Autodesk Inventor part; units mm, degrees
(part 3 of 4)
  line L1598 (-32.17063, 1.012888) -> (-32.17063, -0.001143)
  line L1599 (-32.17063, -0.001143) -> (-32.17063, -0.963359)
  line L1600 (-32.17063, -0.963359) -> (-31.94224, -3.850005)
  line L1601 (-31.94224, -3.850005) -> (-31.272499, -7.565517)
  line L1602 (-31.272499, -7.565517) -> (-30.188344, -11.120628)
  line L1603 (-30.188344, -11.120628) -> (-28.715551, -14.490001)
  line L1604 (-28.715551, -14.490001) -> (-26.883112, -17.647539)
  line L1605 (-26.883112, -17.647539) -> (-24.714784, -20.565161)
  line L1606 (-24.714784, -20.565161) -> (-22.239465, -23.217188)
  line L1607 (-22.239465, -23.217188) -> (-20.201363, -25.028976)
  line L1608 (-20.201363, -25.028976) -> (-19.480987, -25.578797)
  line L1609 (-19.480987, -25.578797) -> (-19.035522, -24.981427)
  line L1610 (-19.035522, -24.981427) -> (-19.739362, -24.443988)
  line L1611 (-19.739362, -24.443988) -> (-21.728906, -22.674586)
  line L1612 (-21.728906, -22.674586) -> (-24.146332, -20.08352)
  line L1613 (-24.146332, -20.08352) -> (-26.262997, -17.234154)
  line L1614 (-26.262997, -17.234154) -> (-28.05202, -14.151102)
  line L1615 (-28.05202, -14.151102) -> (-29.489667, -10.861358)
  line L1616 (-29.489667, -10.861358) -> (-30.547989, -7.388733)
  line L1617 (-30.547989, -7.388733) -> (-31.202243, -3.759899)
  line L1618 (-31.202243, -3.759899) -> (-31.425471, -0.940499)
  line L1619 (-31.425471, -0.940499) -> (-31.425471, -0.001143)
  circle A0 centre (0, 0) radius 38.1
  circle A1 centre (0, 0) radius 38.1
  line L1620 (0, -38.1) -> (0, -50.8)
  line L1621 (0, -38.1) -> (12.7, -38.1) construction
  point P0 (0, 45.086841)
  dimension "d32" = 76.2
  dimension "d33" = 12.7
  dimension "d34" = 90
  constraints: 3244 end point, 1 horizontal, 1 perpendicular, 1 vertical, 1 vertical alignment, 1 other
  measures "d32" distance of L125.end L89.end
  measures "d33" distance of L1620.start L1620.end
  measures "d34" angle of L1620 L1621
sketch "Sketch3 outline for Extrusion2" plane through (0, -45.086841, 3.175) normal (0, 0, 1) x (1, 0, 0)
  circle A0 centre (0, 0) radius 38.1
  line L0 (0.918972, -35.952322) -> (-0.919924, -35.952322)
  line L1 (-0.919924, -35.952322) -> (-3.676459, -35.766299)
  line L2 (-3.676459, -35.766299) -> (-7.246239, -35.221621)
  line L3 (-7.246239, -35.221621) -> (-10.691812, -34.335872)
  line L4 (-10.691812, -34.335872) -> (-13.995083, -33.126655)
  line L5 (-13.995083, -33.126655) -> (-17.136999, -31.612542)
  line L6 (-17.136999, -31.612542) -> (-20.101103, -29.812145)
  line L7 (-20.101103, -29.812145) -> (-22.868896, -27.741982)
  line L8 (-22.868896, -27.741982) -> (-25.421692, -25.421692)
  line L9 (-25.421692, -25.421692) -> (-27.74301, -22.868896)
  line L10 (-27.74301, -22.868896) -> (-29.812145, -20.101103)
  line L11 (-29.812145, -20.101103) -> (-31.612542, -17.136999)
  line L12 (-31.612542, -17.136999) -> (-33.126655, -13.99394)
  line L13 (-33.126655, -13.99394) -> (-34.335872, -10.690669)
  line L14 (-34.335872, -10.690669) -> (-35.221621, -7.246239)
  line L15 (-35.221621, -7.246239) -> (-35.766299, -3.67646)
  line L16 (-35.766299, -3.67646) -> (-35.951293, -0.919925)
  line L17 (-35.951293, -0.919925) -> (-35.951293, 0.918972)
  line L18 (-35.951293, 0.918972) -> (-35.766299, 3.675316)
  line L19 (-35.766299, 3.675316) -> (-35.221621, 7.245096)
  line L20 (-35.221621, 7.245096) -> (-34.335872, 10.689717)
  line L21 (-34.335872, 10.689717) -> (-33.126655, 13.992987)
  line L22 (-33.126655, 13.992987) -> (-31.612542, 17.136046)
  line L23 (-31.612542, 17.136046) -> (-29.812145, 20.100036)
  line L24 (-29.812145, 20.100036) -> (-27.74301, 22.868001)
  line L25 (-27.74301, 22.868001) -> (-25.421692, 25.420701)
  line L26 (-25.421692, 25.420701) -> (-22.868896, 27.740991)
  line L27 (-22.868896, 27.740991) -> (-20.101103, 29.811155)
  line L28 (-20.101103, 29.811155) -> (-17.136999, 31.61157)
  line L29 (-17.136999, 31.61157) -> (-13.995083, 33.125664)
  line L30 (-13.995083, 33.125664) -> (-10.691812, 34.334958)
  line L31 (-10.691812, 34.334958) -> (-7.246239, 35.220592)
  line L32 (-7.246239, 35.220592) -> (-3.676459, 35.765232)
  line L33 (-3.676459, 35.765232) -> (-0.919924, 35.950207)
  line L34 (-0.919924, 35.950207) -> (0.918972, 35.950207)
  line L35 (0.918972, 35.950207) -> (3.675317, 35.765232)
  line L36 (3.675317, 35.765232) -> (7.245096, 35.220592)
  line L37 (7.245096, 35.220592) -> (10.69067, 34.334958)
  line L38 (10.69067, 34.334958) -> (13.99413, 33.125664)
  line L39 (13.99413, 33.125664) -> (17.136999, 31.61157)
  line L40 (17.136999, 31.61157) -> (20.101179, 29.811155)
  line L41 (20.101179, 29.811155) -> (22.868954, 27.740991)
  line L42 (22.868954, 27.740991) -> (25.421653, 25.420701)
  line L43 (25.421653, 25.420701) -> (27.742134, 22.868001)
  line L44 (27.742134, 22.868001) -> (29.812107, 20.100036)
  line L45 (29.812107, 20.100036) -> (31.612332, 17.136046)
  line L46 (31.612332, 17.136046) -> (33.126617, 13.992987)
  line L47 (33.126617, 13.992987) -> (34.33572, 10.689717)
  line L48 (34.33572, 10.689717) -> (35.221545, 7.245096)
  line L49 (35.221545, 7.245096) -> (35.766375, 3.675316)
  line L50 (35.766375, 3.675316) -> (35.952303, 0.918972)
  line L51 (35.952303, 0.918972) -> (35.952303, -0.919925)
  line L52 (35.952303, -0.919925) -> (35.766375, -3.67646)
  line L53 (35.766375, -3.67646) -> (35.221545, -7.246239)
  line L54 (35.221545, -7.246239) -> (34.33572, -10.690669)
  line L55 (34.33572, -10.690669) -> (33.126617, -13.99394)
  line L56 (33.126617, -13.99394) -> (31.612332, -17.136999)
  line L57 (31.612332, -17.136999) -> (29.812107, -20.101103)
  line L58 (29.812107, -20.101103) -> (27.742134, -22.868896)
  line L59 (27.742134, -22.868896) -> (25.421653, -25.421692)
  line L60 (25.421653, -25.421692) -> (22.868954, -27.741982)
  line L61 (22.868954, -27.741982) -> (20.101179, -29.812145)
  line L62 (20.101179, -29.812145) -> (17.136999, -31.612542)
  line L63 (17.136999, -31.612542) -> (13.99413, -33.126655)
  line L64 (13.99413, -33.126655) -> (10.69067, -34.335872)
  line L65 (10.69067, -34.335872) -> (7.245096, -35.221621)
  line L66 (7.245096, -35.221621) -> (3.675317, -35.766299)
  line L67 (3.675317, -35.766299) -> (0.918972, -35.952322)
  line L68 (-29.911357, 16.940403) -> (-28.194667, 16.119919)
  line L69 (-28.194667, 16.119919) -> (-28.483008, 15.517368)
  line L70 (-28.483008, 15.517368) -> (-28.579134, 15.56385)
  line L71 (-28.579134, 15.56385) -> (-29.008045, 15.702534)
  line L72 (-29.008045, 15.702534) -> (-29.370814, 15.721012)
  line L73 (-29.370814, 15.721012) -> (-29.433869, 15.706534)
  line L74 (-29.433869, 15.706534) -> (-29.496906, 15.693199)
  line L75 (-29.496906, 15.693199) -> (-29.769759, 15.530703)
  line L76 (-29.769759, 15.530703) -> (-29.98992, 15.24762)
  line L77 (-29.98992, 15.24762) -> (-30.025048, 15.172182)
  line L78 (-30.025048, 15.172182) -> (-30.05709, 15.103983)
  line L79 (-30.05709, 15.103983) -> (-27.229365, 13.752195)
  line L80 (-27.229365, 13.752195) -> (-27.191094, 13.734478)
  line L81 (-27.191094, 13.734478) -> (-26.930661, 13.63218)
  line L82 (-26.930661, 13.63218) -> (-26.916202, 13.629132)
  line L83 (-26.916202, 13.629132) -> (-26.902753, 13.628179)
  line L84 (-26.902753, 13.628179) -> (-26.792149, 13.661136)
  line L85 (-26.792149, 13.661136) -> (-26.7839, 13.669518)
  line L86 (-26.7839, 13.669518) -> (-26.773556, 13.678662)
  line L87 (-26.773556, 13.678662) -> (-26.665028, 13.817346)
  line L88 (-26.665028, 13.817346) -> (-26.653674, 13.834872)
  line L89 (-26.653674, 13.834872) -> (-26.642301, 13.85335)
  line L90 (-26.642301, 13.85335) -> (-26.462469, 14.188249)
  line L91 (-26.462469, 14.188249) -> (-26.437666, 14.237017)
  line L92 (-26.437666, 14.237017) -> (-25.867157, 13.96384)
  line L93 (-25.867157, 13.96384) -> (-27.129105, 11.324463)
  line L94 (-27.129105, 11.324463) -> (-27.699595, 11.597259)
  line L95 (-27.699595, 11.597259) -> (-27.68306, 11.632311)
  line L96 (-27.68306, 11.632311) -> (-27.552834, 11.935015)
  line L97 (-27.552834, 11.935015) -> (-27.542509, 11.961114)
  line L98 (-27.542509, 11.961114) -> (-27.533194, 11.987974)
  line L99 (-27.533194, 11.987974) -> (-27.474272, 12.213145)
  line L100 (-27.474272, 12.213145) -> (-27.471186, 12.231624)
  line L101 (-27.471186, 12.231624) -> (-27.470157, 12.243054)
  line L102 (-27.470157, 12.243054) -> (-27.514601, 12.347638)
  line L103 (-27.514601, 12.347638) -> (-27.524926, 12.356782)
  line L104 (-27.524926, 12.356782) -> (-27.53527, 12.367069)
  line L105 (-27.53527, 12.367069) -> (-27.772976, 12.503658)
  line L106 (-27.772976, 12.503658) -> (-27.8102, 12.521184)
  line L107 (-27.8102, 12.521184) -> (-27.898039, 12.563475)
  line L108 (-27.898039, 12.563475) -> (-30.645144, 13.877163)
  line L109 (-30.645144, 13.877163) -> (-30.676158, 13.812012)
  line L110 (-30.676158, 13.812012) -> (-30.712334, 13.736574)
  line L111 (-30.712334, 13.736574) -> (-30.750586, 13.066966)
  line L112 (-30.750586, 13.066966) -> (-30.721649, 13.007911)
  line L113 (-30.721649, 13.007911) -> (-30.693722, 12.949999)
  line L114 (-30.693722, 12.949999) -> (-30.075683, 12.431268)
  line L115 (-30.075683, 12.431268) -> (-29.980604, 12.385929)
  line L116 (-29.980604, 12.385929) -> (-30.26584, 11.788521)
  line L117 (-30.26584, 11.788521) -> (-31.98255, 12.609957)
  line L118 (-31.98255, 12.609957) -> (-29.911357, 16.940403)
  line L119 (-9.504426, -27.822582) -> (-10.266045, -29.566152)
  line L120 (-10.266045, -29.566152) -> (-10.876788, -29.29951)
  line L121 (-10.876788, -29.29951) -> (-10.834497, -29.202355)
  line L122 (-10.834497, -29.202355) -> (-10.711434, -28.768281)
  line L123 (-10.711434, -28.768281) -> (-10.704195, -28.404483)
  line L124 (-10.704195, -28.404483) -> (-10.719816, -28.342457)
  line L125 (-10.719816, -28.342457) -> (-10.736199, -28.279401)
  line L126 (-10.736199, -28.279401) -> (-10.90803, -28.01173)
  line L127 (-10.90803, -28.01173) -> (-11.199305, -27.802942)
  line L128 (-11.199305, -27.802942) -> (-11.274742, -27.769871)
  line L129 (-11.274742, -27.769871) -> (-11.344084, -27.739905)
  line L130 (-11.344084, -27.739905) -> (-12.598718, -30.612074)
  line L131 (-12.598718, -30.612074) -> (-12.616243, -30.650307)
  line L132 (-12.616243, -30.650307) -> (-12.708255, -30.915959)
  line L133 (-12.708255, -30.915959) -> (-12.709398, -30.930399)
  line L134 (-12.709398, -30.930399) -> (-12.711303, -30.943848)
  line L135 (-12.711303, -30.943848) -> (-12.674155, -31.053405)
  line L136 (-12.674155, -31.053405) -> (-12.664821, -31.061654)
  line L137 (-12.664821, -31.061654) -> (-12.655486, -31.070969)
  line L138 (-12.655486, -31.070969) -> (-12.51604, -31.174315)
  line L139 (-12.51604, -31.174315) -> (-12.496419, -31.185688)
  line L140 (-12.496419, -31.185688) -> (-12.47775, -31.196013)
  line L141 (-12.47775, -31.196013) -> (-12.136755, -31.364511)
  line L142 (-12.136755, -31.364511) -> (-12.087034, -31.388266)
  line L143 (-12.087034, -31.388266) -> (-12.339256, -31.967043)
  line L144 (-12.339256, -31.967043) -> (-15.021306, -30.797068)
  line L145 (-15.021306, -30.797068) -> (-14.769084, -30.217262)
  line L146 (-14.769084, -30.217262) -> (-14.734032, -30.23174)
  line L147 (-14.734032, -30.23174) -> (-14.425994, -30.351622)
  line L148 (-14.425994, -30.351622) -> (-14.399133, -30.360937)
  line L149 (-14.399133, -30.360937) -> (-14.373225, -30.369186)
  line L150 (-14.373225, -30.369186) -> (-14.145958, -30.420888)
  line L151 (-14.145958, -30.420888) -> (-14.126337, -30.422964)
  line L152 (-14.126337, -30.422964) -> (-14.114907, -30.423993)
  line L153 (-14.114907, -30.423993) -> (-14.012608, -30.376444)
  line L154 (-14.012608, -30.376444) -> (-14.003274, -30.3661)
  line L155 (-14.003274, -30.3661) -> (-13.993939, -30.354746)
  line L156 (-13.993939, -30.354746) -> (-13.865733, -30.111859)
  line L157 (-13.865733, -30.111859) -> (-13.84935, -30.074654)
  line L158 (-13.84935, -30.074654) -> (-13.809916, -29.984719)
  line L159 (-13.809916, -29.984719) -> (-12.591478, -27.195247)
  line L160 (-12.591478, -27.195247) -> (-12.656629, -27.16631)
  line L161 (-12.656629, -27.16631) -> (-12.734163, -27.13221)
  line L162 (-12.734163, -27.13221) -> (-13.405866, -27.117732)
  line L163 (-13.405866, -27.117732) -> (-13.462825, -27.148746)
  line L164 (-13.462825, -27.148746) -> (-13.520547, -27.178711)
  line L165 (-13.520547, -27.178711) -> (-14.017752, -27.812257)
  line L166 (-14.017752, -27.812257) -> (-14.05909, -27.909412)
  line L167 (-14.05909, -27.909412) -> (-14.66469, -27.645855)
  line L168 (-14.66469, -27.645855) -> (-13.903071, -25.901256)
  line L169 (-13.903071, -25.901256) -> (-9.504426, -27.822582)
  line L170 (5.837492, -31.82855) -> (6.61035, -31.72728)
  line L171 (6.61035, -31.72728) -> (6.626923, -31.895739)
  line L172 (6.626923, -31.895739) -> (6.568059, -32.634688)
  line L173 (6.568059, -32.634688) -> (6.313742, -33.231049)
  line L174 (6.313742, -33.231049) -> (6.234303, -33.329213)
  line L175 (6.234303, -33.329213) -> (6.153722, -33.426368)
  line L176 (6.153722, -33.426368) -> (5.610034, -33.802587)
  line L177 (5.610034, -33.802587) -> (4.875276, -34.029968)
  line L178 (4.875276, -34.029968) -> (4.700587, -34.053723)
  line L179 (4.700587, -34.053723) -> (4.502087, -34.079574)
  line L180 (4.502087, -34.079574) -> (3.60807, -34.017566)
  line L181 (3.60807, -34.017566) -> (2.845308, -33.700269)
  line L182 (2.845308, -33.700269) -> (2.711958, -33.59898)
  line L183 (2.711958, -33.59898) -> (2.578608, -33.496682)
  line L184 (2.578608, -33.496682) -> (2.072259, -32.844505)
  line L185 (2.072259, -32.844505) -> (1.781747, -32.000114)
  line L186 (1.781747, -32.000114) -> (1.756029, -31.802699)
  line L187 (1.756029, -31.802699) -> (1.742504, -31.703486)
  line L188 (1.742504, -31.703486) -> (1.777746, -30.802269)
  line L189 (1.777746, -30.802269) -> (1.79832, -30.720621)
  line L190 (1.79832, -30.720621) -> (1.817941, -30.638953)
  line L191 (1.817941, -30.638953) -> (2.190941, -29.877258)
  line L192 (2.190941, -29.877258) -> (2.245805, -29.806944)
  line L193 (2.245805, -29.806944) -> (2.298764, -29.739774)
  line L194 (2.298764, -29.739774) -> (2.906268, -29.215804)
  line L195 (2.906268, -29.215804) -> (2.97542, -29.178561)
  line L196 (2.97542, -29.178561) -> (3.043809, -29.140328)
  line L197 (3.043809, -29.140328) -> (3.861245, -28.891249)
  line L198 (3.861245, -28.891249) -> (3.956304, -28.879876)
  line L199 (3.956304, -28.879876) -> (4.022408, -28.870599)
  line L200 (4.022408, -28.870599) -> (4.659059, -28.884029)
  line L201 (4.659059, -28.884029) -> (4.720209, -28.896412)
  line L202 (4.720209, -28.896412) -> (4.780979, -28.907784)
  line L203 (4.780979, -28.907784) -> (5.382768, -29.13105)
  line L204 (5.382768, -29.13105) -> (5.442395, -29.164121)
  line L205 (5.442395, -29.164121) -> (5.537645, -28.756908)
  line L206 (5.537645, -28.756908) -> (6.206299, -28.66905)
  line L207 (6.206299, -28.66905) -> (6.469952, -30.662728)
  line L208 (6.469952, -30.662728) -> (5.753671, -30.757806)
  line L209 (5.753671, -30.757806) -> (5.731955, -30.651374)
  line L210 (5.731955, -30.651374) -> (5.564505, -30.19867)
  line L211 (5.564505, -30.19867) -> (5.315522, -29.854493)
  line L212 (5.315522, -29.854493) -> (5.253228, -29.801801)
  line L213 (5.253228, -29.801801) -> (5.190363, -29.74909)
  line L214 (5.190363, -29.74909) -> (4.837938, -29.581659)
  line L215 (4.837938, -29.581659) -> (4.431792, -29.543426)
  line L216 (4.431792, -29.543426) -> (4.342829, -29.555808)
  line L217 (4.342829, -29.555808) -> (4.244721, -29.56821)
  line L218 (4.244721, -29.56821) -> (3.835337, -29.747032)
  line L219 (3.835337, -29.747032) -> (3.533585, -30.077759)
  line L220 (3.533585, -30.077759) -> (3.490151, -30.166628)
  line L221 (3.490151, -30.166628) -> (3.445574, -30.255534)
  line L222 (3.445574, -30.255534) -> (3.320796, -30.787791)
  line L223 (3.320796, -30.787791) -> (3.322892, -31.437872)
  line L224 (3.322892, -31.437872) -> (3.342513, -31.585662)
  line L225 (3.342513, -31.585662) -> (3.362135, -31.735528)
  line L226 (3.362135, -31.735528) -> (3.528441, -32.372198)
  line L227 (3.528441, -32.372198) -> (3.785997, -32.854849)
  line L228 (3.785997, -32.854849) -> (3.850958, -32.929239)
  line L229 (3.850958, -32.929239) -> (3.914966, -33.002639)
  line L230 (3.914966, -33.002639) -> (4.293489, -33.241374)
  line L231 (4.293489, -33.241374) -> (4.741926, -33.305458)
  line L232 (4.741926, -33.305458) -> (4.843272, -33.292028)
  line L233 (4.843272, -33.292028) -> (4.927854, -33.280674)
  line L234 (4.927854, -33.280674) -> (5.291709, -33.145247)
  line L235 (5.291709, -33.145247) -> (5.572887, -32.901369)
  line L236 (5.572887, -32.901369) -> (5.617083, -32.837285)
  line L237 (5.617083, -32.837285) -> (5.660707, -32.772172)
  line L238 (5.660707, -32.772172) -> (5.803392, -32.390791)
  line L239 (5.803392, -32.390791) -> (5.843588, -31.931896)
  line L240 (5.843588, -31.931896) -> (5.837492, -31.82855)
  line L241 (7.072313, 28.470416) -> (6.501956, 28.644342)
  line L242 (7.366064, 28.755975) -> (7.072313, 28.470416)
  line L243 (7.401115, 28.710446) -> (7.366064, 28.755975)
  line L244 (7.888795, 28.28163) -> (7.401115, 28.710446)
  line L245 (7.952041, 28.241053) -> (7.888795, 28.28163)
  line L246 (8.013954, 28.202001) -> (7.952041, 28.241053)
  line L247 (8.685657, 27.89282) -> (8.013954, 28.202001)
  line L248 (8.758238, 27.87015) -> (8.685657, 27.89282)
  line L249 (8.90797, 27.824621) -> (8.758238, 27.87015)
  line L250 (9.596437, 27.727465) -> (8.90797, 27.824621)
  line L251 (10.202037, 27.807095) -> (9.596437, 27.727465)
  line L252 (10.311575, 27.849576) -> (10.202037, 27.807095)
  line L253 (10.42016, 27.891867) -> (10.311575, 27.849576)
  line L254 (10.856214, 28.217241) -> (10.42016, 27.891867)
  line L255 (11.144441, 28.691586) -> (10.856214, 28.217241)
  line L256 (11.180826, 28.808553) -> (11.144441, 28.691586)
  line L257 (11.210734, 28.908947) -> (11.180826, 28.808553)
  line L258 (11.25093, 29.377957) -> (11.210734, 28.908947)
  line L259 (11.143488, 29.811155) -> (11.25093, 29.377957)
  line L260 (11.100054, 29.891736) -> (11.143488, 29.811155)
  line L261 (11.055667, 29.97327) -> (11.100054, 29.891736)
  line L262 (10.212324, 30.749557) -> (11.055667, 29.97327)
  line L263 (10.088309, 30.824043) -> (10.212324, 30.749557)
  line L264 (10.056304, 30.843474) -> (10.088309, 30.824043)
  line L265 (9.621012, 31.091695) -> (10.056304, 30.843474)
  line L266 (9.566339, 31.121604) -> (9.621012, 31.091695)
  line L267 (9.420416, 31.202376) -> (9.566339, 31.121604)
  line L268 (8.939974, 31.571184) -> (9.420416, 31.202376)
  line L269 (8.787003, 31.901892) -> (8.939974, 31.571184)
  line L270 (8.805672, 31.9619) -> (8.787003, 31.901892)
  line L271 (8.818054, 32.00419) -> (8.805672, 31.9619)
  line L272 (9.09085, 32.284416) -> (8.818054, 32.00419)
  line L273 (9.133332, 32.297751) -> (9.09085, 32.284416)
  line L274 (9.174671, 32.312229) -> (9.133332, 32.297751)
  line L275 (9.678924, 32.292607) -> (9.174671, 32.312229)
  line L276 (9.737979, 32.273938) -> (9.678924, 32.292607)
  line L277 (9.836086, 32.24403) -> (9.737979, 32.273938)
  line L278 (10.250424, 32.036194) -> (9.836086, 32.24403)
  line L279 (10.561701, 31.752159) -> (10.250424, 32.036194)
  line L280 (10.609326, 31.683769) -> (10.561701, 31.752159)
  line L281 (10.655617, 31.61557) -> (10.609326, 31.683769)
  line L282 (10.807636, 30.8229) -> (10.655617, 31.61557)
  line L283 (10.792015, 30.732984) -> (10.807636, 30.8229)
  line L284 (11.437239, 30.535626) -> (10.792015, 30.732984)
  line L285 (11.963209, 32.259651) -> (11.437239, 30.535626)
  line L286 (11.379136, 32.43853) -> (11.963209, 32.259651)
  line L287 (11.137392, 32.148018) -> (11.379136, 32.43853)
  line L288 (11.104245, 32.1945) -> (11.137392, 32.148018)
  line L289 (10.671238, 32.596455) -> (11.104245, 32.1945)
  line L290 (10.61847, 32.630554) -> (10.671238, 32.596455)
  line L291 (10.564749, 32.664654) -> (10.61847, 32.630554)
  line L292 (9.914763, 32.953071) -> (10.564749, 32.664654)
  line L293 (9.839325, 32.97574) -> (9.914763, 32.953071)
  line L294 (9.686163, 33.022413) -> (9.839325, 32.97574)
  line L295 (8.994839, 33.124521) -> (9.686163, 33.022413)
  line L296 (8.401621, 33.053274) -> (8.994839, 33.124521)
  line L297 (8.29818, 33.012888) -> (8.401621, 33.053274)
  line L298 (8.193786, 32.973645) -> (8.29818, 33.012888)
  line L299 (7.776401, 32.654367) -> (8.193786, 32.973645)
  line L300 (7.492937, 32.176783) -> (7.776401, 32.654367)
  line L301 (7.456932, 32.056959) -> (7.492937, 32.176783)
  line L302 (7.440359, 32.005333) -> (7.456932, 32.056959)
  line L303 (7.398068, 31.499937) -> (7.440359, 32.005333)
  line L304 (7.405116, 31.450216) -> (7.398068, 31.499937)
  line L305 (7.412545, 31.401829) -> (7.405116, 31.450216)
  line L306 (7.598473, 30.940629) -> (7.412545, 31.401829)
  line L307 (7.629525, 30.897195) -> (7.598473, 30.940629)
  line L308 (7.652195, 30.864238) -> (7.629525, 30.897195)
  line L309 (7.976616, 30.528387) -> (7.652195, 30.864238)
  line L310 (8.018145, 30.494287) -> (7.976616, 30.528387)
  line L311 (8.059483, 30.46114) -> (8.018145, 30.494287)
  line L312 (8.37457, 30.244161) -> (8.059483, 30.46114)
  line L313 (8.836533, 29.960887) -> (8.37457, 30.244161)
  line L314 (8.951405, 29.893641) -> (8.836533, 29.960887)
  line L315 (8.962835, 29.887545) -> (8.951405, 29.893641)
  line L316 (9.12495, 29.793438) -> (8.962835, 29.887545)
  line L317 (9.146667, 29.781246) -> (9.12495, 29.793438)
  line L318 (9.27716, 29.705617) -> (9.146667, 29.781246)
  line L319 (9.70388, 29.339857) -> (9.27716, 29.705617)
  line L320 (9.827895, 28.987432) -> (9.70388, 29.339857)
  line L321 (9.807131, 28.919233) -> (9.827895, 28.987432)
  line L322 (9.793795, 28.875799) -> (9.807131, 28.919233)
  line L323 (9.500045, 28.590621) -> (9.793795, 28.875799)
  line L324 (9.500045, 28.590621) -> (9.409366, 28.56357)
  line L325 (8.848916, 28.596717) -> (9.409366, 28.56357)
  line L326 (8.782812, 28.616338) -> (8.848916, 28.596717)
  line L327 (8.685657, 28.646437) -> (8.782812, 28.616338)
  line L328 (8.273605, 28.86437) -> (8.685657, 28.646437)
  line L329 (7.956042, 29.176408) -> (8.273605, 28.86437)
  line L330 (7.907655, 29.25318) -> (7.956042, 29.176408)
  line L331 (7.857935, 29.330332) -> (7.907655, 29.25318)
  line L332 (7.685341, 30.207966) -> (7.857935, 29.330332)
  line L333 (7.69982, 30.306264) -> (7.685341, 30.207966)
  line L334 (7.068312, 30.498478) -> (7.69982, 30.306264)
  line L335 (6.501956, 28.644342) -> (7.068312, 30.498478)
  line L336 (14.207871, 25.663588) -> (13.702474, 25.979628)
  line L337 (14.56563, 25.863042) -> (14.207871, 25.663588)
  line L338 (14.587347, 25.810273) -> (14.56563, 25.863042)
  line L339 (14.94682, 25.267729) -> (14.587347, 25.810273)
  line L340 (14.997684, 25.212865) -> (14.94682, 25.267729)
  line L341 (15.047214, 25.158192) -> (14.997684, 25.212865)
  line L342 (15.614713, 24.684799) -> (15.047214, 25.158192)
  line L343 (15.678722, 24.644604) -> (15.614713, 24.684799)
  line L344 (15.810929, 24.561737) -> (15.678722, 24.644604)
  line L345 (16.450818, 24.288941) -> (15.810929, 24.561737)
  line L346 (17.05737, 24.208359) -> (16.450818, 24.288941)
  line L347 (17.174147, 24.220741) -> (17.05737, 24.208359)
  line L348 (17.289971, 24.234267) -> (17.174147, 24.220741)
  line L349 (17.794224, 24.43372) -> (17.289971, 24.234267)
  line L350 (18.197322, 24.816054) -> (17.794224, 24.43372)
  line L351 (18.262283, 24.919495) -> (18.197322, 24.816054)
  line L352 (18.317147, 25.008459) -> (18.262283, 24.919495)
  line L353 (18.487835, 25.898284) -> (18.317147, 25.008459)
  line L354 (18.46707, 25.987057) -> (18.487835, 25.898284)
  line L355 (18.445353, 26.077164) -> (18.46707, 25.987057)
  line L356 (18.218849, 26.546175) -> (18.445353, 26.077164)
  line L357 (17.832324, 27.045475) -> (18.218849, 26.546175)
  line L358 (17.731359, 27.149679) -> (17.832324, 27.045475)
  line L359 (17.705451, 27.17673) -> (17.731359, 27.149679)
  line L360 (17.350931, 27.530107) -> (17.705451, 27.17673)
  line L361 (17.306354, 27.573541) -> (17.350931, 27.530107)
  line L362 (17.186529, 27.689175) -> (17.306354, 27.573541)
  line L363 (16.818483, 28.170949) -> (17.186529, 27.689175)
  line L364 (16.75657, 28.52947) -> (16.818483, 28.170949)
  line L365 (16.79067, 28.582049) -> (16.75657, 28.52947)
  line L366 (16.81353, 28.619386) -> (16.79067, 28.582049)
  line L367 (17.149191, 28.819983) -> (16.81353, 28.619386)
  line L368 (17.193768, 28.822078) -> (17.149191, 28.819983)
  line L369 (17.237012, 28.825126) -> (17.193768, 28.822078)
  line L370 (17.719929, 28.675203) -> (17.237012, 28.825126)
  line L371 (17.772507, 28.642247) -> (17.719929, 28.675203)
  line L372 (17.859375, 28.587382) -> (17.772507, 28.642247)
  line L373 (18.432018, 27.922728) -> (17.859375, 28.587382)
  line L374 (18.460022, 27.844242) -> (18.432018, 27.922728)
  line L375 (18.486692, 27.766708) -> (18.460022, 27.844242)
  line L376 (18.426875, 26.961655) -> (18.486692, 27.766708)
  line L377 (18.387441, 26.878978) -> (18.426875, 26.961655)
  line L378 (18.960084, 26.520267) -> (18.387441, 26.878978)
  line L379 (19.916966, 28.047886) -> (18.960084, 26.520267)
  line L380 (19.399187, 28.372308) -> (19.916966, 28.047886)
  line L381 (19.090196, 28.154376) -> (19.399187, 28.372308)
  line L382 (19.070574, 28.208097) -> (19.090196, 28.154376)
  line L383 (18.75663, 28.710446) -> (19.070574, 28.208097)
  line L384 (18.713958, 28.757118) -> (18.75663, 28.710446)
  line L385 (18.670524, 28.804362) -> (18.713958, 28.757118)
  line L386 (18.118646, 29.249941) -> (18.670524, 28.804362)
  line L387 (18.05178, 29.292232) -> (18.118646, 29.249941)
  line L388 (17.916335, 29.377005) -> (18.05178, 29.292232)
  line L389 (17.276445, 29.65723) -> (17.916335, 29.377005)
  line L390 (16.685514, 29.742955) -> (17.276445, 29.65723)
  line L391 (16.574834, 29.730382) -> (16.685514, 29.742955)
  line L392 (16.463201, 29.719143) -> (16.574834, 29.730382)
  line L393 (15.976283, 29.519499) -> (16.463201, 29.719143)
  line L394 (15.579471, 29.132022) -> (15.976283, 29.519499)
  line L395 (15.513367, 29.026676) -> (15.579471, 29.132022)
  line L396 (15.484221, 28.981146) -> (15.513367, 29.026676)
  line L397 (15.310675, 28.503562) -> (15.484221, 28.981146)
  line L398 (15.305532, 28.454033) -> (15.310675, 28.503562)
  line L399 (15.299245, 28.405455) -> (15.305532, 28.454033)
  line L400 (15.359253, 27.912441) -> (15.299245, 28.405455)
  line L401 (15.376779, 27.863101) -> (15.359253, 27.912441)
  line L402 (15.390305, 27.823668) -> (15.376779, 27.863101)
  line L403 (15.615666, 27.414283) -> (15.390305, 27.823668)
  line L404 (15.64767, 27.37085) -> (15.615666, 27.414283)
  line L405 (15.678722, 27.328558) -> (15.64767, 27.37085)
  line L406 (15.927705, 27.037284) -> (15.678722, 27.328558)
  line L407 (16.299561, 26.642187) -> (15.927705, 27.037284)
  line L408 (16.392716, 26.54827) -> (16.299561, 26.642187)
  line L409 (16.392716, 26.54827) -> (16.534257, 26.406729)
  line L410 (16.552164, 26.389013) -> (16.534257, 26.406729)
  line L411 (16.658463, 26.282713) -> (16.552164, 26.389013)
  line L412 (16.974693, 25.817513) -> (16.658463, 26.282713)
  line L413 (17.002697, 25.445466) -> (16.974693, 25.817513)
  line L414 (16.965359, 25.384315) -> (17.002697, 25.445466)
  line L415 (16.940403, 25.346215) -> (16.965359, 25.384315)
  line L416 (16.583025, 25.147905) -> (16.940403, 25.346215)
  line L417 (16.5354, 25.145809) -> (16.583025, 25.147905)
  line L418 (16.487775, 25.144666) -> (16.5354, 25.145809)
  line L419 (15.956852, 25.322403) -> (16.487775, 25.144666)
  line L420 (15.897797, 25.358788) -> (15.956852, 25.322403)
  line L421 (15.812072, 25.412509) -> (15.897797, 25.358788)
  line L422 (15.471076, 25.730644) -> (15.812072, 25.412509)
  line L423 (15.245524, 26.115264) -> (15.471076, 25.730644)
  line L424 (15.218855, 26.201942) -> (15.245524, 26.115264)
  line L425 (15.190851, 26.288809) -> (15.218855, 26.201942)
  line L426 (15.252001, 27.18073) -> (15.190851, 26.288809)
  line L427 (15.292197, 27.271599) -> (15.252001, 27.18073)
  line L428 (14.731937, 27.623071) -> (15.292197, 27.271599)
  line L429 (13.702474, 25.979628) -> (14.731937, 27.623071)
  line L430 (25.152096, 15.362491) -> (25.731788, 15.649575)
  line L431 (25.731788, 15.649575) -> (25.852755, 15.404782)
  line L432 (25.852755, 15.404782) -> (25.873329, 15.362491)
  line L433 (25.873329, 15.362491) -> (26.062495, 15.11427)
  line L434 (26.062495, 15.11427) -> (26.080022, 15.107221)
  line L435 (26.080022, 15.107221) -> (26.096595, 15.100744)
  line L436 (26.096595, 15.100744) -> (26.392251, 15.172182)
  line L437 (26.392251, 15.172182) -> (26.434542, 15.192946)
  line L438 (26.434542, 15.192946) -> (28.930663, 16.430053)
  line L439 (28.930663, 16.430053) -> (28.972954, 16.45177)
  line L440 (28.972954, 16.45177) -> (29.209556, 16.644937)
  line L441 (29.209556, 16.644937) -> (29.214699, 16.661701)
  line L442 (29.214699, 16.661701) -> (29.219081, 16.679037)
  line L443 (29.219081, 16.679037) -> (29.134117, 16.979836)
  line L444 (29.134117, 16.979836) -> (29.113353, 17.022318)
  line L445 (29.113353, 17.022318) -> (28.992576, 17.267301)
  line L446 (28.992576, 17.267301) -> (29.571505, 17.554575)
  line L447 (29.571505, 17.554575) -> (31.73749, 13.185838)
  line L448 (31.73749, 13.185838) -> (30.052899, 12.350686)
  line L449 (30.052899, 12.350686) -> (29.765625, 12.929425)
  line L450 (29.765625, 12.929425) -> (29.82468, 12.970573)
  line L451 (29.82468, 12.970573) -> (30.258639, 13.319188)
  line L452 (30.258639, 13.319188) -> (30.2855, 13.347001)
  line L453 (30.2855, 13.347001) -> (30.312169, 13.375957)
  line L454 (30.312169, 13.375957) -> (30.488954, 13.668375)
  line L455 (30.488954, 13.668375) -> (30.498479, 13.697521)
  line L456 (30.498479, 13.697521) -> (30.507813, 13.72743)
  line L457 (30.507813, 13.72743) -> (30.513909, 14.058138)
  line L458 (30.513909, 14.058138) -> (30.50667, 14.094333)
  line L459 (30.50667, 14.094333) -> (30.498479, 14.130337)
  line L460 (30.498479, 14.130337) -> (30.252543, 14.726793)
  line L461 (30.252543, 14.726793) -> (30.211204, 14.80947)
  line L462 (30.211204, 14.80947) -> (29.92774, 15.382113)
  line L463 (29.92774, 15.382113) -> (28.67006, 14.758797)
  line L464 (28.67006, 14.758797) -> (28.723971, 14.649259)
  line L465 (28.723971, 14.649259) -> (28.753879, 14.588299)
  line L466 (28.753879, 14.588299) -> (29.072205, 14.235874)
  line L467 (29.072205, 14.235874) -> (29.106305, 14.22673)
  line L468 (29.106305, 14.22673) -> (29.139261, 14.218158)
  line L469 (29.139261, 14.218158) -> (29.656087, 14.346555)
  line L470 (29.656087, 14.346555) -> (29.726382, 14.380654)
  line L471 (29.726382, 14.380654) -> (30.001274, 13.827633)
  line L472 (30.001274, 13.827633) -> (27.983878, 12.826936)
  line L473 (27.983878, 12.826936) -> (27.712988, 13.382053)
  line L474 (27.712988, 13.382053) -> (27.788425, 13.422249)
  line L475 (27.788425, 13.422249) -> (28.236101, 13.770673)
  line L476 (28.236101, 13.770673) -> (28.250388, 13.800582)
  line L477 (28.250388, 13.800582) -> (28.263913, 13.831633)
  line L478 (28.263913, 13.831633) -> (28.176093, 14.29893)
  line L479 (28.176093, 14.29893) -> (28.145041, 14.361795)
  line L480 (28.145041, 14.361795) -> (28.090368, 14.471332)
  line L481 (28.090368, 14.471332) -> (26.666, 13.764387)
  line L482 (26.666, 13.764387) -> (26.95975, 13.173265)
  line L483 (26.95975, 13.173265) -> (27.019567, 13.052488)
  line L484 (27.019567, 13.052488) -> (27.323606, 12.595479)
  line L485 (27.323606, 12.595479) -> (27.634501, 12.337161)
  line L486 (27.634501, 12.337161) -> (27.697557, 12.314491)
  line L487 (27.697557, 12.314491) -> (27.760612, 12.292774)
  line L488 (27.760612, 12.292774) -> (28.176093, 12.289726)
  line L489 (28.176093, 12.289726) -> (28.724733, 12.429363)
  line L490 (28.724733, 12.429363) -> (28.855225, 12.47775)
  line L491 (28.855225, 12.47775) -> (29.1425, 11.899201)
  line L492 (29.1425, 11.899201) -> (27.319224, 10.994707)
  line L493 (27.319224, 10.994707) -> (25.152096, 15.362491)
  line L494 (19.891439, 21.741384) -> (20.367688, 22.178391)
  line L495 (20.367688, 22.178391) -> (20.551712, 21.977032)
  line L496 (20.551712, 21.977032) -> (20.583716, 21.94198)
  line L497 (20.583716, 21.94198) -> (20.834795, 21.756624)
  line L498 (20.834795, 21.756624) -> (20.853464, 21.754909)
  line L499 (20.853464, 21.754909) -> (20.87118, 21.752623)
  line L500 (20.87118, 21.752623) -> (21.135785, 21.902547)
  line L501 (21.135785, 21.902547) -> (21.170836, 21.934551)
  line L502 (21.170836, 21.934551) -> (23.224236, 23.815738)
  line L503 (23.224236, 23.815738) -> (23.259479, 23.848695)
  line L504 (23.259479, 23.848695) -> (23.433024, 24.098821)
  line L505 (23.433024, 24.098821) -> (23.433024, 24.116157)
  line L506 (23.433024, 24.116157) -> (23.432262, 24.135016)
  line L507 (23.432262, 24.135016) -> (23.268813, 24.400764)
  line L508 (23.268813, 24.400764) -> (23.236809, 24.435626)
  line L509 (23.236809, 24.435626) -> (23.052786, 24.636222)
  line L510 (23.052786, 24.636222) -> (23.529417, 25.072467)
  line L511 (23.529417, 25.072467) -> (26.82221, 21.476779)
  line L512 (26.82221, 21.476779) -> (25.434036, 20.206525)
  line L513 (25.434036, 20.206525) -> (24.997791, 20.682966)
  line L514 (24.997791, 20.682966) -> (25.043321, 20.739925)
  line L515 (25.043321, 20.739925) -> (25.362598, 21.194458)
  line L516 (25.362598, 21.194458) -> (25.381458, 21.229701)
  line L517 (25.381458, 21.229701) -> (25.398984, 21.264753)
  line L518 (25.398984, 21.264753) -> (25.4889, 21.594508)
  line L519 (25.4889, 21.594508) -> (25.490043, 21.624417)
  line L520 (25.490043, 21.624417) -> (25.490043, 21.656611)
  line L521 (25.490043, 21.656611) -> (25.404318, 21.97608)
  line L522 (25.404318, 21.97608) -> (25.386602, 22.008084)
  line L523 (25.386602, 22.008084) -> (25.369076, 22.04104)
  line L524 (25.369076, 22.04104) -> (24.96693, 22.545484)
  line L525 (24.96693, 22.545484) -> (24.905018, 22.613683)
  line L526 (24.905018, 22.613683) -> (24.473916, 23.08498)
  line L527 (24.473916, 23.08498) -> (23.438358, 22.137243)
  line L528 (23.438358, 22.137243) -> (23.520083, 22.047136)
  line L529 (23.520083, 22.047136) -> (23.565422, 21.997797)
  line L530 (23.565422, 21.997797) -> (23.96852, 21.74748)
  line L531 (23.96852, 21.74748) -> (24.003762, 21.74748)
  line L532 (24.003762, 21.74748) -> (24.037862, 21.748432)
  line L533 (24.037862, 21.748432) -> (24.500967, 22.015132)
  line L534 (24.500967, 22.015132) -> (24.558688, 22.067901)
  line L535 (24.558688, 22.067901) -> (24.975312, 21.612225)
  line L536 (24.975312, 21.612225) -> (23.314343, 20.091844)
  line L537 (23.314343, 20.091844) -> (22.900958, 20.549616)
  line L538 (22.900958, 20.549616) -> (22.96287, 20.608671)
  line L539 (22.96287, 20.608671) -> (23.295673, 21.068538)
  line L540 (23.295673, 21.068538) -> (23.300817, 21.101494)
  line L541 (23.300817, 21.101494) -> (23.305008, 21.134641)
  line L542 (23.305008, 21.134641) -> (23.092029, 21.558313)
  line L543 (23.092029, 21.558313) -> (23.044595, 21.610129)
  line L544 (23.044595, 21.610129) -> (22.960775, 21.700045)
  line L545 (22.960775, 21.700045) -> (21.789009, 20.626197)
  line L546 (21.789009, 20.626197) -> (22.234208, 20.139279)
  line L547 (22.234208, 20.139279) -> (22.325267, 20.040028)
  line L548 (22.325267, 20.040028) -> (22.744938, 19.685508)
  line L549 (22.744938, 19.685508) -> (23.114889, 19.523392)
  line L550 (23.114889, 19.523392) -> (23.181945, 19.519011)
  line L551 (23.181945, 19.519011) -> (23.248239, 19.516153)
  line L552 (23.248239, 19.516153) -> (23.647146, 19.628929)
  line L553 (23.647146, 19.628929) -> (24.137112, 19.915251)
  line L554 (24.137112, 19.915251) -> (24.248555, 19.997737)
  line L555 (24.248555, 19.997737) -> (24.685943, 19.520154)
  line L556 (24.685943, 19.520154) -> (23.18404, 18.145696)
  line L557 (23.18404, 18.145696) -> (19.891439, 21.741384)
  line L558 (-1.875853, 29.406151) -> (-1.860232, 30.051946)
  line L559 (-1.860232, 30.051946) -> (-1.587436, 30.04585)
  line L560 (-1.587436, 30.04585) -> (-1.539811, 30.044707)
  line L561 (-1.539811, 30.044707) -> (-1.231963, 30.096333)
  line L562 (-1.231963, 30.096333) -> (-1.217676, 30.107763)
  line L563 (-1.217676, 30.107763) -> (-1.20415, 30.120145)
  line L564 (-1.20415, 30.120145) -> (-1.129855, 30.414658)
  line L565 (-1.129855, 30.414658) -> (-1.128712, 30.46114)
  line L566 (-1.128712, 30.46114) -> (-1.060513, 33.246441)
  line L567 (-1.060513, 33.246441) -> (-1.05937, 33.295209)
  line L568 (-1.05937, 33.295209) -> (-1.119188, 33.594865)
  line L569 (-1.119188, 33.594865) -> (-1.13157, 33.606295)
  line L570 (-1.13157, 33.606295) -> (-1.145095, 33.618678)
  line L571 (-1.145095, 33.618678) -> (-1.451038, 33.683829)
  line L572 (-1.451038, 33.683829) -> (-1.498663, 33.684972)
  line L573 (-1.498663, 33.684972) -> (-1.770316, 33.69202)
  line L574 (-1.770316, 33.69202) -> (-1.754886, 34.337815)
  line L575 (-1.754886, 34.337815) -> (3.119247, 34.217991)
  line L576 (3.119247, 34.217991) -> (3.073718, 32.337184)
  line L577 (3.073718, 32.337184) -> (2.42678, 32.353568)
  line L578 (2.42678, 32.353568) -> (2.418588, 32.425957)
  line L579 (2.418588, 32.425957) -> (2.311908, 32.971549)
  line L580 (2.311908, 32.971549) -> (2.299526, 33.007744)
  line L581 (2.299526, 33.007744) -> (2.286191, 33.045082)
  line L582 (2.286191, 33.045082) -> (2.11055, 33.339595)
  line L583 (2.11055, 33.339595) -> (2.088832, 33.360169)
  line L584 (2.088832, 33.360169) -> (2.066163, 33.383029)
  line L585 (2.066163, 33.383029) -> (1.776603, 33.542097)
  line L586 (1.776603, 33.542097) -> (1.741551, 33.551622)
  line L587 (1.741551, 33.551622) -> (1.705166, 33.561909)
  line L588 (1.705166, 33.561909) -> (1.063561, 33.622678)
  line L589 (1.063561, 33.622678) -> (0.97155, 33.624774)
  line L590 (0.97155, 33.624774) -> (0.332804, 33.640395)
  line L591 (0.332804, 33.640395) -> (0.298704, 32.236791)
  line L592 (0.298704, 32.236791) -> (0.420624, 32.233743)
  line L593 (0.420624, 32.233743) -> (0.48787, 32.2326)
  line L594 (0.48787, 32.2326) -> (0.947737, 32.350519)
  line L595 (0.947737, 32.350519) -> (0.97155, 32.375284)
  line L596 (0.97155, 32.375284) -> (0.994219, 32.401192)
  line L597 (0.994219, 32.401192) -> (1.122426, 32.917828)
  line L598 (1.122426, 32.917828) -> (1.124522, 32.995362)
  line L599 (1.124522, 32.995362) -> (1.742504, 32.980884)
  line L600 (1.742504, 32.980884) -> (1.686687, 30.729936)
  line L601 (1.686687, 30.729936) -> (1.069658, 30.748605)
  line L602 (1.069658, 30.748605) -> (1.069658, 30.83433)
  line L603 (1.069658, 30.83433) -> (0.969455, 31.3944)
  line L604 (0.969455, 31.3944) -> (0.949833, 31.420308)
  line L605 (0.949833, 31.420308) -> (0.929259, 31.446978)
  line L606 (0.929259, 31.446978) -> (0.474345, 31.586805)
  line L607 (0.474345, 31.586805) -> (0.404051, 31.587757)
  line L608 (0.404051, 31.587757) -> (0.28213, 31.590805)
  line L609 (0.28213, 31.590805) -> (0.242888, 30.001273)
  line L610 (0.242888, 30.001273) -> (0.903351, 29.9847)
  line L611 (0.903351, 29.9847) -> (1.038796, 29.981461)
  line L612 (1.038796, 29.981461) -> (1.585341, 30.038421)
  line L613 (1.585341, 30.038421) -> (1.958531, 30.192345)
  line L614 (1.958531, 30.192345) -> (2.007108, 30.237874)
  line L615 (2.007108, 30.237874) -> (2.055876, 30.283404)
  line L616 (2.055876, 30.283404) -> (2.252091, 30.649354)
  line L617 (2.252091, 30.649354) -> (2.384489, 31.20028)
  line L618 (2.384489, 31.20028) -> (2.401824, 31.33744)
  line L619 (2.401824, 31.33744) -> (3.048, 31.3222)
  line L620 (3.048, 31.3222) -> (2.99828, 29.286898)
  line L621 (2.99828, 29.286898) -> (-1.875853, 29.406151)
  line L622 (-23.801127, 17.377791) -> (-24.286902, 17.804701)
  line L623 (-24.286902, 17.804701) -> (-24.107051, 18.009108)
  line L624 (-24.107051, 18.009108) -> (-24.076057, 18.045303)
  line L625 (-24.076057, 18.045303) -> (-23.917904, 18.332767)
  line L626 (-23.917904, 18.332767) -> (-23.918951, 18.351246)
  line L627 (-23.918951, 18.351246) -> (-24.097755, 18.597372)
  line L628 (-24.097755, 18.597372) -> (-24.132883, 18.628233)
  line L629 (-24.132883, 18.628233) -> (-26.226821, 20.465034)
  line L630 (-26.226821, 20.465034) -> (-26.262997, 20.497038)
  line L631 (-26.262997, 20.497038) -> (-26.531697, 20.64277)
  line L632 (-26.531697, 20.64277) -> (-26.54928, 20.639532)
  line L633 (-26.54928, 20.639532) -> (-26.566863, 20.637436)
  line L634 (-26.566863, 20.637436) -> (-26.813847, 20.445222)
  line L635 (-26.813847, 20.445222) -> (-26.84486, 20.409217)
  line L636 (-26.84486, 20.409217) -> (-27.023663, 20.20443)
  line L637 (-27.023663, 20.20443) -> (-27.510467, 20.630388)
  line L638 (-27.510467, 20.630388) -> (-24.29618, 24.296179)
  line L639 (-24.29618, 24.296179) -> (-22.881298, 23.056024)
  line L640 (-22.881298, 23.056024) -> (-23.307084, 22.570249)
  line L641 (-23.307084, 22.570249) -> (-23.368083, 22.610445)
  line L642 (-23.368083, 22.610445) -> (-23.855915, 22.878288)
  line L643 (-23.855915, 22.878288) -> (-23.892091, 22.891814)
  line L644 (-23.892091, 22.891814) -> (-23.929296, 22.906101)
  line L645 (-23.929296, 22.906101) -> (-24.267243, 22.958679)
  line L646 (-24.267243, 22.958679) -> (-24.297208, 22.955821)
  line L647 (-24.297208, 22.955821) -> (-24.328222, 22.953726)
  line L648 (-24.328222, 22.953726) -> (-24.636222, 22.832758)
  line L649 (-24.636222, 22.832758) -> (-24.666207, 22.811041)
  line L650 (-24.666207, 22.811041) -> (-24.697182, 22.790467)
  line L651 (-24.697182, 22.790467) -> (-25.155049, 22.336696)
  line L652 (-25.155049, 22.336696) -> (-25.216028, 22.266211)
  line L653 (-25.216028, 22.266211) -> (-25.636671, 21.786913)
  line L654 (-25.636671, 21.786913) -> (-24.581434, 20.860893)
  line L655 (-24.581434, 20.860893) -> (-24.500834, 20.952523)
  line L656 (-24.500834, 20.952523) -> (-24.45639, 21.00453)
  line L657 (-24.45639, 21.00453) -> (-24.251755, 21.43125)
  line L658 (-24.251755, 21.43125) -> (-24.255889, 21.465349)
  line L659 (-24.255889, 21.465349) -> (-24.261051, 21.500592)
  line L660 (-24.261051, 21.500592) -> (-24.576272, 21.93055)
  line L661 (-24.576272, 21.93055) -> (-24.635193, 21.981033)
  line L662 (-24.635193, 21.981033) -> (-24.227981, 22.446234)
  line L663 (-24.227981, 22.446234) -> (-22.535064, 20.962239)
  line L664 (-22.535064, 20.962239) -> (-22.945382, 20.499895)
  line L665 (-22.945382, 20.499895) -> (-23.011524, 20.555712)
  line L666 (-23.011524, 20.555712) -> (-23.5045, 20.83708)
  line L667 (-23.5045, 20.83708) -> (-23.53757, 20.838033)
  line L668 (-23.53757, 20.838033) -> (-23.570641, 20.839176)
  line L669 (-23.570641, 20.839176) -> (-23.969586, 20.579524)
  line L670 (-23.969586, 20.579524) -> (-24.016106, 20.525803)
  line L671 (-24.016106, 20.525803) -> (-24.095678, 20.433792)
  line L672 (-24.095678, 20.433792) -> (-22.899891, 19.386042)
  line L673 (-22.899891, 19.386042) -> (-22.46477, 19.882866)
  line L674 (-22.46477, 19.882866) -> (-22.375901, 19.985355)
  line L675 (-22.375901, 19.985355) -> (-22.068949, 20.441221)
  line L676 (-22.068949, 20.441221) -> (-21.949048, 20.82565)
  line L677 (-21.949048, 20.82565) -> (-21.952134, 20.891754)
  line L678 (-21.952134, 20.891754) -> (-21.956287, 20.959)
  line L679 (-21.956287, 20.959) -> (-22.111316, 21.344382)
  line L680 (-22.111316, 21.344382) -> (-22.449282, 21.799296)
  line L681 (-22.449282, 21.799296) -> (-22.543313, 21.900261)
  line L682 (-22.543313, 21.900261) -> (-22.117507, 22.386036)
  line L683 (-22.117507, 22.386036) -> (-20.586859, 21.043582)
  line L684 (-20.586859, 21.043582) -> (-23.801127, 17.377791)
  line L685 (-7.424737, -33.519408) -> (-7.334059, -32.879633)
  line L686 (-7.334059, -32.879633) -> (-7.064121, -32.917905)
  line L687 (-7.064121, -32.917905) -> (-7.016686, -32.924096)
  line L688 (-7.016686, -32.924096) -> (-6.704457, -32.907561)
  line L689 (-6.704457, -32.907561) -> (-6.688836, -32.898245)
  line L690 (-6.688836, -32.898245) -> (-6.674549, -32.88792)
  line L691 (-6.674549, -32.88792) -> (-6.565963, -32.604742)
  line L692 (-6.565963, -32.604742) -> (-6.558725, -32.558222)
  line L693 (-6.558725, -32.558222) -> (-6.168961, -29.799724)
  line L694 (-6.168961, -29.799724) -> (-6.162865, -29.752176)
  line L695 (-6.162865, -29.752176) -> (-6.187821, -29.447299)
  line L696 (-6.187821, -29.447299) -> (-6.199251, -29.433869)
  line L697 (-6.199251, -29.433869) -> (-6.211633, -29.42042)
  line L698 (-6.211633, -29.42042) -> (-6.506146, -29.319131)
  line L699 (-6.506146, -29.319131) -> (-6.553771, -29.312959)
  line L700 (-6.553771, -29.312959) -> (-6.823329, -29.274687)
  line L701 (-6.823329, -29.274687) -> (-6.73227, -28.63495)
  line L702 (-6.73227, -28.63495) -> (-1.904809, -29.318102)
  line L703 (-1.904809, -29.318102) -> (-2.169414, -31.181573)
  line L704 (-2.169414, -31.181573) -> (-2.809113, -31.09061)
  line L705 (-2.809113, -31.09061) -> (-2.809113, -30.924208)
  line L706 (-2.809113, -30.924208) -> (-2.850261, -30.463255)
  line L707 (-2.850261, -30.463255) -> (-2.858833, -30.425022)
  line L708 (-2.858833, -30.425022) -> (-2.868168, -30.386788)
  line L709 (-2.868168, -30.386788) -> (-3.008566, -30.075683)
  line L710 (-3.008566, -30.075683) -> (-3.027045, -30.051908)
  line L711 (-3.027045, -30.051908) -> (-3.046857, -30.027105)
  line L712 (-3.046857, -30.027105) -> (-3.316605, -29.834872)
  line L713 (-3.316605, -29.834872) -> (-3.350704, -29.821422)
  line L714 (-3.350704, -29.821422) -> (-3.384804, -29.806944)
  line L715 (-3.384804, -29.806944) -> (-4.016311, -29.671575)
  line L716 (-4.016311, -29.671575) -> (-4.10718, -29.659174)
  line L717 (-4.10718, -29.659174) -> (-4.73983, -29.570286)
  line L718 (-4.73983, -29.570286) -> (-4.937189, -30.960384)
  line L719 (-4.937189, -30.960384) -> (-4.816221, -30.976919)
  line L720 (-4.816221, -30.976919) -> (-4.748975, -30.986235)
  line L721 (-4.748975, -30.986235) -> (-4.27882, -30.923179)
  line L722 (-4.27882, -30.923179) -> (-4.251769, -30.901481)
  line L723 (-4.251769, -30.901481) -> (-4.226243, -30.878736)
  line L724 (-4.226243, -30.878736) -> (-4.039171, -30.37953)
  line L725 (-4.039171, -30.37953) -> (-4.027741, -30.302016)
  line L726 (-4.027741, -30.302016) -> (-3.415855, -30.387817)
  line L727 (-3.415855, -30.387817) -> (-3.731895, -32.617124)
  line L728 (-3.731895, -32.617124) -> (-4.342828, -32.527208)
  line L729 (-4.342828, -32.527208) -> (-4.332541, -32.441445)
  line L730 (-4.332541, -32.441445) -> (-4.367784, -31.87507)
  line L731 (-4.367784, -31.87507) -> (-4.384167, -31.847161)
  line L732 (-4.384167, -31.847161) -> (-4.401883, -31.818205)
  line L733 (-4.401883, -31.818205) -> (-4.837938, -31.62702)
  line L734 (-4.837938, -31.62702) -> (-4.90728, -31.617704)
  line L735 (-4.90728, -31.617704) -> (-5.028057, -31.60014)
  line L736 (-5.028057, -31.60014) -> (-5.25037, -33.175232)
  line L737 (-5.25037, -33.175232) -> (-4.596003, -33.267225)
  line L738 (-4.596003, -33.267225) -> (-4.462653, -33.285836)
  line L739 (-4.462653, -33.285836) -> (-3.914013, -33.292028)
  line L740 (-3.914013, -33.292028) -> (-3.525393, -33.183519)
  line L741 (-3.525393, -33.183519) -> (-3.471672, -33.144219)
  line L742 (-3.471672, -33.144219) -> (-3.417951, -33.103928)
  line L743 (-3.417951, -33.103928) -> (-3.180207, -32.762857)
  line L744 (-3.180207, -32.762857) -> (-2.983611, -32.231628)
  line L745 (-2.983611, -32.231628) -> (-2.950655, -32.097269)
  line L746 (-2.950655, -32.097269) -> (-2.310955, -32.187166)
  line L747 (-2.310955, -32.187166) -> (-2.596134, -34.203589)
  line L748 (-2.596134, -34.203589) -> (-7.424737, -33.519408)
  line L749 (-19.514058, 26.962608) -> (-19.53888, 27.003184)
  line L750 (-19.53888, 27.003184) -> (-19.754869, 27.21483)
  line L751 (-19.754869, 27.21483) -> (-19.772452, 27.217878)
  line L752 (-19.772452, 27.217878) -> (-19.791045, 27.221116)
  line L753 (-19.791045, 27.221116) -> (-20.087673, 27.107388)
  line L754 (-20.087673, 27.107388) -> (-20.127963, 27.08148)
  line L755 (-20.127963, 27.08148) -> (-20.346029, 26.942986)
  line L756 (-20.346029, 26.942986) -> (-20.691234, 27.489722)
  line L757 (-20.691234, 27.489722) -> (-18.695479, 28.747593)
  line L758 (-18.695479, 28.747593) -> (-15.261145, 26.846974)
  line L759 (-15.261145, 26.846974) -> (-16.523017, 28.848939)
  line L760 (-16.523017, 28.848939) -> (-16.547782, 28.889325)
  line L761 (-16.547782, 28.889325) -> (-16.763809, 29.10097)
  line L762 (-16.763809, 29.10097) -> (-16.781336, 29.104209)
  line L763 (-16.781336, 29.104209) -> (-16.800004, 29.107257)
  line L764 (-16.800004, 29.107257) -> (-17.096613, 28.993528)
  line L765 (-17.096613, 28.993528) -> (-17.136999, 28.967621)
  line L766 (-17.136999, 28.967621) -> (-17.3736, 28.817887)
  line L767 (-17.3736, 28.817887) -> (-17.717833, 29.364432)
  line L768 (-17.717833, 29.364432) -> (-15.813024, 30.565534)
  line L769 (-15.813024, 30.565534) -> (-15.46879, 30.018799)
  line L770 (-15.46879, 30.018799) -> (-15.663101, 29.895736)
  line L771 (-15.663101, 29.895736) -> (-15.704439, 29.870209)
  line L772 (-15.704439, 29.870209) -> (-15.934944, 29.652849)
  line L773 (-15.934944, 29.652849) -> (-15.940087, 29.63437)
  line L774 (-15.940087, 29.63437) -> (-15.945231, 29.616844)
  line L775 (-15.945231, 29.616844) -> (-15.84598, 29.331475)
  line L776 (-15.84598, 29.331475) -> (-15.821215, 29.29128)
  line L777 (-15.821215, 29.29128) -> (-13.762482, 26.0263)
  line L778 (-13.762482, 26.0263) -> (-15.043976, 25.218962)
  line L779 (-15.043976, 25.218962) -> (-18.71091, 27.243786)
  line L780 (-18.71091, 27.243786) -> (-17.326165, 25.048654)
  line L781 (-17.326165, 25.048654) -> (-17.30121, 25.009221)
  line L782 (-17.30121, 25.009221) -> (-17.087278, 24.796432)
  line L783 (-17.087278, 24.796432) -> (-17.0688, 24.793385)
  line L784 (-17.0688, 24.793385) -> (-17.051083, 24.790146)